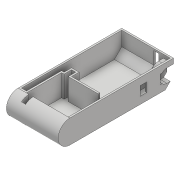
# Autodesk Inventor part: leg_hind_upper
Saved by Autodesk Inventor 2017 (Build 210142000, 142)
## iProperties
Created: 2019-03-28
Part Number: leg_hind_upper
Material: Generic
Document SubType Name: Modeling
Designer: mfans
Density: 1 g/cm^3
Appearance: Default
Author: mfans
Autodesk Inventor part; units mm, degrees
ref_plane "YZ Plane" through (0, 0, 0) normal (1, 0, 0) x (0, 1, 0)
ref_plane "XZ Plane" through (0, 0, 0) normal (0, 1, 0) x (-1, 0, 0)
ref_plane "XY Plane" through (0, 0, 0) normal (0, 0, 1) x (1, 0, 0)
sketch "Sketch1" plane through (0, 0, 0) normal (0, 0, 1) x (1, 0, 0)
  line L0 (15.5, -34.5227) -> (-15.5, -34.5227)
  line L1 (-15.5, -34.5227) -> (-15.5, 34.5227)
  line L2 (-15.5, 34.5227) -> (15.5, 34.5227)
  line L3 (15.5, 34.5227) -> (15.5, -34.5227)
  line L4 (15.5, -34.5227) -> (-15.5, 34.5227) construction
  line L5 (-15.5, -34.5227) -> (15.5, 34.5227) construction
  point P0 (0, 0)
  dimension "d0" = 31
  constraints: 12 end point, 2 midpoint, 2 parallel, 1 horizontal, 1 perpendicular
  measures "d0" distance between parallel lines of L1 L3
extrude "Extrusion1" add sketch "Sketch1" along normal blind 14
fillet "Fillet1" radius 7 2 edges at (0, -34.5227, 14) (0, -34.5227, 0)
sketch "Sketch2" plane through (0, 0, 14) normal (0, 0, 1) x (1, 0, 0)
  line L0 (14.5, -27.5227) -> (-10.5, -27.5227)
  line L1 (-10.5, -27.5227) -> (-10.5, -6.5252)
  line L2 (-10.5, -6.5252) -> (14.5, -6.5252)
  line L3 (14.5, -6.5252) -> (14.5, -27.5227)
  line L4 (15.5, -27.5227) -> (-15.5, -27.5227) projected
  line L5 (15.5, -27.5227) -> (15.5, 34.5227) projected
  point P0 (0, 0)
  dimension "d4" = 25
  dimension "d5" = 0
  dimension "d6" = 1
  constraints: 8 end point, 2 parallel, 1 horizontal, 1 perpendicular
  measures "d4" distance of L1.end L2.end
  measures "d5" distance between parallel lines of L4 L0
  measures "d6" distance between parallel lines of L3 L5
extrude "Extrusion2" cut sketch "Sketch2" against normal blind 13
sketch "Sketch3" plane through (0, 0, 14) normal (0, 0, 1) x (1, 0, 0)
  line L0 (-9, -2.0252) -> (-6.5, -2.0252)
  line L1 (-6.5, -2.0252) -> (-6.5, -32.0227)
  line L2 (-6.5, -32.0227) -> (-9, -32.0227)
  line L3 (-9, -32.0227) -> (-9, -2.0252)
  line L4 (14.5, -6.5252) -> (14.5, -27.5227) projected
  line L5 (-10.5, -6.5252) -> (14.5, -6.5252) projected
  line L6 (14.5, -27.5227) -> (-10.5, -27.5227) projected
  point P0 (0, 0)
  dimension "d9" = 21
  dimension "d10" = 4.5
  dimension "d11" = 4.5
  dimension "d12" = 2.5
  constraints: 8 end point, 2 parallel, 1 horizontal, 1 perpendicular
  measures "d9" distance between parallel lines of L4 L1
  measures "d10" distance between parallel lines of L5 L0
  measures "d11" distance between parallel lines of L6 L2
  measures "d12" distance between parallel lines of L1 L3
extrude "Extrusion3" cut sketch "Sketch3" against normal up to surface (13 mm away) contours L0 L1 L5 L3 | L5 L1 L6 L3 | L6 L1 L2 L3
sketch "Sketch4" plane through (0, 0, 1) normal (0, 0, 1) x (1, 0, 0)
  line L0 (14.5, -27.5227) -> (-6.5, -27.5227) projected
  line L1 (14.5, -6.5252) -> (14.5, -27.5227) projected
  line L2 (-6.5, -6.5252) -> (14.5, -6.5252) projected
  line L3 (-6.5, -6.5252) -> (-6.5, -2.0252) projected
  line L4 (-6.5, -2.0252) -> (-9, -2.0252) projected
  line L5 (-9, -2.0252) -> (-9, -6.5252) projected
  line L6 (-10.5, -6.5252) -> (-9, -6.5252) projected
  line L7 (-10.5, -27.5227) -> (-10.5, -6.5252) projected
  line L8 (-9, -27.5227) -> (-10.5, -27.5227) projected
  line L9 (-9, -27.5227) -> (-9, -31.1283) projected
  line L10 (-6.5, -31.1283) -> (-9, -31.1283) projected
  line L11 (-6.5, -31.1283) -> (-6.5, -27.5227) projected
  line L12 (-6.5, -27.5227) -> (-9, -27.5227)
  line L13 (-9, -27.5227) -> (-9, -31.1283)
  line L14 (-9, -31.1283) -> (-6.5, -31.1283)
  line L15 (-6.5, -31.1283) -> (-6.5, -27.5227)
  point P0 (0, 0)
  constraints: 8 end point, 2 parallel, 1 horizontal, 1 perpendicular
extrude "Extrusion4" cut sketch "Sketch4" along normal mid plane 13 contours L11 L10 L9 L12
sketch "Sketch5" plane through (15.5, 34.5227, 14) normal (1, 0, 0) x (0, 0, -1)
  arc A0 (0, -62.0455) -> (14, -62.0455) centre (7, -62.0455) ccw projected
  line L0 (14, 0) -> (14, -62.0455) projected
  line L1 (14, 0) -> (0, 0) projected
  line L2 (0, -62.0455) -> (0, 0) projected
  line L3 (9.75, -4) -> (4.25, -4)
  line L4 (4.25, -4) -> (4.25, -20)
  line L5 (4.25, -20) -> (9.75, -20)
  line L6 (9.75, -20) -> (9.75, -4)
  line L7 (9.75, -4) -> (4.25, -20) construction
  line L8 (4.25, -4) -> (9.75, -20) construction
  circle A1 centre (7, -4) radius 4
  line L9 (14, 0) -> (0, 0) projected
  line L10 (3, -4) -> (11, -4)
  line L11 (11, -4) -> (11, 0)
  line L12 (11, 0) -> (3, 0)
  line L13 (3, 0) -> (3, -4)
  point P0 (14, -34.5227)
  point P1 (7, -12)
  dimension "d18" = 8
  dimension "d17" = 4
  dimension "d19" = 5.5
  dimension "d20" = 7
  dimension "d21" = 16
  constraints: 20 end point, 4 parallel, 3 midpoint, 2 horizontal, 2 perpendicular, 1 horizontal alignment, 1 point on line, 2 other
  measures "d17" distance between parallel lines of L1 L3
  measures "d19" distance of L4.end L5.end
  measures "d20" distance from line of L2 point (7, -4)
  measures "d21" distance of L5.end L3.start
extrude "Extrusion5" cut sketch "Sketch5" against normal blind 4 contours L1 A1 L13 | L11 A1 L1 | A1 L10 L3 | L10 L4 A1 | A1 L6 L10 | L4 L3 L6 A1
extrude "Extrusion6" cut sketch "Sketch5" against normal blind 3 contours A1 L6 L5 L4 | L4 L3 L6 A1
sketch "Sketch6" plane through (15.5, -27.5227, 0) normal (1, 0, 0) x (0, 0, -1)
  line L0 (-9.75, 42.0455) -> (-9.75, 55.1407) projected
  line L1 (-4.25, 46.0455) -> (-9.75, 46.0455)
  line L2 (-9.75, 46.0455) -> (-9.75, 54.0455)
  line L3 (-9.75, 54.0455) -> (-4.25, 54.0455)
  line L4 (-4.25, 54.0455) -> (-4.25, 46.0455)
  line L5 (-4.25, 55.1407) -> (-4.25, 42.0455) projected
  line L6 (-4.25, 42.0455) -> (-9.75, 42.0455) projected
  point P0 (0, 27.5227)
  dimension "d26" = 0
  dimension "d27" = 4
  dimension "d28" = 8
  constraints: 8 end point, 2 parallel, 1 horizontal, 1 perpendicular, 1 point on line
  measures "d26" distance between parallel lines of L5 L4
  measures "d27" distance between parallel lines of L6 L1
  measures "d28" distance of L3.end L1.start
extrude "Extrusion7" add sketch "Sketch6" against normal blind 1 contours L0 L3 L4 L1
chamfer "Chamfer1" distance 5 angle 45 1 edges at (0, 34.5227, 0)
sketch "Sketch7" plane through (0, 0, 14) normal (0, 0, 1) x (1, 0, 0)
  line L0 (-15.5, -27.5227) -> (-9, -27.5227) projected
  line L1 (-10.5, -27.5227) -> (-10.5, -6.5252) projected
  line L2 (-15.5, -27.5227) -> (-10.5, -27.5227)
  line L3 (-10.5, -27.5227) -> (-10.5, -26.5227)
  line L4 (-10.5, -26.5227) -> (-15.5, -26.5227)
  line L5 (-15.5, -26.5227) -> (-15.5, -27.5227)
  point P0 (0, 0)
  dimension "d34" = 1
  constraints: 8 end point, 2 parallel, 1 horizontal, 1 perpendicular, 1 point on line
  measures "d34" distance between parallel lines of L0 L4
extrude "Extrusion8" add sketch "Sketch7" along normal blind 1
sketch "Sketch8" plane through (0, 0, 14) normal (0, 0, 1) x (1, 0, 0)
  line L0 (14.5, -27.5227) -> (-6.5, -27.5227) projected
  line L1 (15.5, 29.5227) -> (15.5, -27.5227) projected
  line L2 (14.5, -27.5227) -> (15.5, -27.5227)
  line L3 (15.5, -27.5227) -> (15.5, -26.5227)
  line L4 (15.5, -26.5227) -> (14.5, -26.5227)
  line L5 (14.5, -26.5227) -> (14.5, -27.5227)
  point P0 (0, 0)
  dimension "d37" = 1
  constraints: 8 end point, 2 parallel, 1 horizontal, 1 perpendicular, 1 point on line
  measures "d37" distance between parallel lines of L2 L4
extrude "Extrusion9" add sketch "Sketch8" along normal blind 1
shell "Shell1" thickness 1 removed faces 1 at (-2.1667, 22.3401, 14)
sketch "Sketch9" plane through (0, 0, 14) normal (0, 0, 1) x (1, 0, 0)
  line L0 (-6.5, -6.5252) -> (14.5, -6.5252) projected
  line L1 (-5.5, -5.5252) -> (14.5, -5.5252) projected
  line L2 (14.5, -6.5252) -> (11.5, -6.5252)
  line L3 (11.5, -6.5252) -> (11.5, -5.5252)
  line L4 (11.5, -5.5252) -> (14.5, -5.5252)
  line L5 (14.5, -5.5252) -> (14.5, -6.5252)
  point P0 (0, 0)
  dimension "d41" = 3
  constraints: 8 end point, 2 parallel, 1 horizontal, 1 perpendicular, 1 point on line
  measures "d41" distance of L3.end L4.end
extrude "Extrusion10" cut sketch "Sketch9" against normal up to surface (13 mm away)
sketch "Sketch10" plane through (0, 0, 15) normal (0, 0, 1) x (1, 0, 0)
  line L0 (-15.5, -27.5227) -> (-10.5, -27.5227) projected
  line L1 (-10.5, -27.5227) -> (-10.5, -26.5227) projected
  line L2 (-10.5, -26.5227) -> (-15.5, -26.5227) projected
  line L3 (-15.5, -26.5227) -> (-15.5, -27.5227) projected
  line L4 (14.5, -27.5227) -> (15.5, -27.5227) projected
  line L5 (15.5, -27.5227) -> (15.5, -26.5227) projected
  line L6 (15.5, -26.5227) -> (14.5, -26.5227) projected
  line L7 (14.5, -26.5227) -> (14.5, -27.5227) projected
  point P0 (0, 0)
extrude "Extrusion11" cut sketch "Sketch10" against normal blind 1
sketch "Sketch11" plane through (-14.5, 33.5227, 14) normal (0, -1, 0) x (1, 0, 0)
  line L0 (19.1427, -1) -> (22.1427, -1)
  line L1 (22.1427, -1) -> (22.1427, -13)
  line L2 (22.1427, -13) -> (19.1427, -13)
  line L3 (19.1427, -13) -> (19.1427, -1)
  line L4 (19.1427, -1) -> (22.1427, -13) construction
  line L5 (22.1427, -1) -> (19.1427, -13) construction
  line L6 (0, 0) -> (29, 0) projected
  point P0 (14.5, -14)
  point P1 (20.6427, -7)
  dimension "d46" = 3
  dimension "d47" = 12
  dimension "d48" = 1
  constraints: 12 end point, 2 midpoint, 2 parallel, 1 horizontal, 1 perpendicular
  measures "d46" distance of L0.start L0.end
  measures "d47" distance of L0.end L1.end
  measures "d48" distance between parallel lines of L6 L0
extrude "Extrusion12" cut sketch "Sketch11" along normal mid plane 10
body "Solid1"
